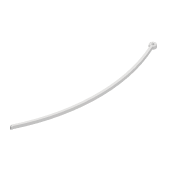
# Autodesk Inventor part: Part_13
Saved by Autodesk Inventor 2022 (Build 260153000, 153)
## iProperties
Created: 2022-05-03
Part Number: Part_13
Material: Generic
Document SubType Name: Modeling
Designer: dell
Density: 1 g/cm^3
Appearance: Default
Author: dell
Autodesk Inventor part; units mm, degrees
ref_plane "YZ Plane" through (0, 0, 0) normal (1, 0, 0) x (0, 1, 0)
ref_plane "XZ Plane" through (0, 0, 0) normal (0, 1, 0) x (-1, 0, 0)
ref_plane "XY Plane" through (0, 0, 0) normal (0, 0, 1) x (1, 0, 0)
sketch "Sketch1" plane through (0, 0, 0) normal (0, 1, 0) x (-1, 0, 0)
  line L0 (0, 0) -> (0, -521.938) construction
  line L1 (-4, 0) -> (-4, -521.938)
  line L2 (4, -521.938) -> (4, 0)
  arc A0 (4, 0) -> (-4, 0) centre (0, 0) ccw
  arc A1 (-4, -521.938) -> (4, -521.938) centre (0, -521.938) ccw
  circle A2 centre (0, 0) radius 1.5
  circle A3 centre (0, -521.938) radius 1.5
  arc A4 (-4, -3) -> (-4, -518.938) centre (537.7121, -260.969) ccw
  arc A5 (4, -3) -> (4, -518.938) centre (545.7121, -260.969) ccw
  point P0 (0, -260.969)
  point P1 (-4, -501.4199)
  point P2 (-4, -20.5181)
  dimension "d0" = 8
  dimension "d1" = 521.938
  dimension "d2" = 3
  dimension "d3" = 3
  dimension "d24" = 600
  dimension "d25" = 600
  dimension "d26" = 3
  dimension "d27" = 3
  constraints: 8 end point, 8 point on circle, 6 centre point, 4 point on line, 4 tangent, 2 coincident, 2 horizontal alignment, 1 midpoint, 1 parallel, 1 vertical
  measures "d0" diameter of A1
  measures "d1" distance of L0.end L0.start
  measures "d2" diameter of A2
  measures "d3" diameter of A3
  measures "d24" radius of A4
  measures "d25" radius of A5
  measures "d26" vertical distance of L0.start A4.start
  measures "d27" vertical distance of A4.end L0.end
extrude "Extrusion1" add sketch "Sketch1" along normal blind 10 contours A0 L2 A5 L1 | L1 A5 A4 | L1 A5 L2 A1
sketch "Sketch5" plane through (0, 10, 0) normal (0, 1, 0) x (1, 0, 0)
  arc A0 (4, 3) -> (4, 518.938) centre (-537.7121, 260.969) ccw projected
  line L0 (4, 518.938) -> (4, 521.938) projected
  arc A1 (4, 521.938) -> (-4, 521.938) centre (0, 521.938) ccw projected
  line L1 (-4, 521.938) -> (-4, 518.938) projected
  arc A2 (-4, 3) -> (-4, 518.938) centre (-545.7121, 260.969) ccw projected
  line L2 (-4, 3) -> (-4, 0) projected
  arc A3 (-4, 0) -> (4, 0) centre (0, 0) ccw projected
  line L3 (4, 0) -> (4, 3) projected
  circle A4 centre (0, 521.938) radius 1.5 projected
  circle A5 centre (0, 0) radius 1.5 projected
  circle A6 centre (0, 521.938) radius 11
  point P0 (6.6919, 513.2076)
  point P1 (-0.2637, 510.9412)
  dimension "d45" = 22
  constraints: 1 centre point, 1 coincident
  measures "d45" diameter of A6
extrude "Extrusion5" add sketch "Sketch5" against normal blind 10 contours A0 L0 A1 L1 A2 A6 picked at (6.2374, 520.1049)
sketch "Sketch6" plane through (0, 10, 0) normal (0, 1, 0) x (1, 0, 0)
  arc A0 (4, 3) -> (6.6919, 513.2076) centre (-537.7121, 260.969) ccw projected
  arc A1 (6.6919, 513.2076) -> (-0.2637, 510.9412) centre (0, 521.938) ccw projected
  arc A2 (-4, 3) -> (-0.2637, 510.9412) centre (-545.7121, 260.969) ccw projected
  line L0 (-4, 3) -> (-4, 0) projected
  arc A3 (-4, 0) -> (4, 0) centre (0, 0) ccw projected
  line L1 (4, 0) -> (4, 3) projected
  circle A4 centre (0, 521.938) radius 1.5 projected
  circle A5 centre (0, 0) radius 1.5 projected
  circle A6 centre (0, 529.938) radius 1.1
  circle A7 centre (0, 521.938) radius 4.25
  dimension "d48" = 2.2
  dimension "d49" = 8
  dimension "d55" = 8.5
  constraints: 2 centre point, 1 coincident, 1 vertical alignment
  measures "d48" diameter of A6
  measures "d49" distance of A1.centre A6.centre
  measures "d55" diameter of A7
extrude "Extrusion6" cut sketch "Sketch6" against normal blind 100 contours A4 | A6 | A7
pattern_circular "Circular Pattern1" count 8 over 360 about axis through (0, 0, -521.938) along (0, 1, 0) of "Extrusion6"
sketch "Sketch2" plane through (0, 10, 0) normal (0, 1, 0) x (1, 0, 0)
  arc A0 (4, 3) -> (6.6919, 513.2076) centre (-537.7121, 260.969) ccw projected
  arc A1 (-4, 3) -> (-0.2637, 510.9412) centre (-545.7121, 260.969) ccw projected
  line L0 (-4, 3) -> (-4, 0) projected
  arc A2 (-4, 0) -> (4, 0) centre (0, 0) ccw projected
  line L1 (4, 0) -> (4, 3) projected
  circle A3 centre (0, 0) radius 1.5 projected
  arc A4 (-4, 3) -> (-4, 518.938) centre (-545.7121, 260.969) ccw projected
  line L2 (54.2879, 260.969) -> (58.1281, 268.7691)
  line L3 (58.1281, 268.7691) -> (62.2796, 257.8034)
  arc A5 (4, 3) -> (4, 518.938) centre (-537.7121, 260.969) ccw projected
  arc A6 (6.6919, 513.2076) -> (-0.2637, 510.9412) centre (0, 521.938) ccw projected
  constraints: 4 end point, 3 point on circle
extrude "Extrusion2" [suppressed]
body "Solid1"
